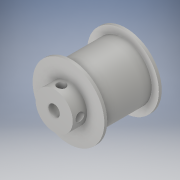
# Autodesk Inventor part: Timing Belt - 8mm Bore 5mm Pitch 14 Teeth 15mm Wide
Saved by Autodesk Inventor 2017 SP1 (Build 210196100, 196)
## iProperties
Created: 2017-10-06
Part Number: Timing Belt - 8mm Bore 5mm Pitch 14 Teeth 15mm Wide
Material: Aluminum 6061
Document SubType Name: Modeling
Designer: Zach
Density: 2.7 g/cm^3
Appearance: Aluminum - Flat
Author: Zach
Autodesk Inventor part; units mm, degrees
ref_plane "YZ Plane" through (0, 0, 0) normal (1, 0, 0) x (0, 1, 0)
ref_plane "XZ Plane" through (0, 0, 0) normal (0, 1, 0) x (-1, 0, 0)
ref_plane "XY Plane" through (0, 0, 0) normal (0, 0, 1) x (1, 0, 0)
sketch "Sketch1" plane through (0, 0, 0) normal (0, 0, 1) x (1, 0, 0)
  circle A0 centre (0, 0) radius 12.5
  circle A1 centre (0, 0) radius 2
  dimension "d0" = 25
  dimension "d1" = 4
  constraints: 2 centre point, 2 coincident
  measures "d0" diameter of A0
  measures "d1" diameter of A1
extrude "Extrusion1" add sketch "Sketch1" along normal blind 20
sketch "Sketch2" plane through (0, 0, 20) normal (0, 0, 1) x (1, 0, 0)
  circle A0 centre (0, 0) radius 2 projected
  circle A1 centre (0, 0) radius 6.5
  dimension "d4" = 13
  constraints: 1 centre point, 1 coincident
  measures "d4" diameter of A1
extrude "Extrusion2" add sketch "Sketch2" along normal blind 5
ref_plane "Work Plane1" through (0, 0, 10) normal (0, 0, -1) x (-1, 0, 0)
sketch "Sketch3" plane through (0, 0, 10) normal (0, 0, -1) x (-1, 0, 0)
  circle A0 centre (0, 0) radius 10
  circle A1 centre (0, 0) radius 12.5 projected
  dimension "d7" = 20
  constraints: 1 centre point, 1 coincident
  measures "d7" diameter of A0
extrude "Extrusion3" cut sketch "Sketch3" along normal mid plane 18
sketch "Sketch6" plane through (0, 0, 0) normal (0, 1, 0) x (-1, 0, 0)
  line L0 (6.5, 25) -> (-6.5, 25) projected
  line L1 (-6.5, 20) -> (6.5, 20) projected
  line L2 (-2, 25) -> (2, 25) projected
  line L3 (-2, 25) -> (2, 25) projected
  line L4 (2, 0) -> (-2, 0) projected
  circle A0 centre (0, 22.5) radius 1.5
  line L5 (6.5, 20) -> (6.5, 25) projected
  line L6 (-6.5, 20) -> (-6.5, 25) projected
  point P0 (0, 0)
  point P1 (0, 20)
  point P2 (6.5, 22.5)
  dimension "d36" = 3
  constraints: 2 midpoint, 1 centre point, 1 horizontal alignment, 1 vertical alignment
  measures "d36" diameter of A0
extrude "Extrusion4" cut sketch "Sketch6" along normal through all contours A0
sketch "Sketch7" plane through (0, 0, 0) normal (1, 0, 0) x (0, 1, 0)
  line L0 (-2, 25) -> (2, 25) projected
  line L1 (6.5, 20) -> (6.5, 25) projected
  circle A0 centre (0, 22.5) radius 1.5
  point P0 (0, 0)
  point P1 (0, 25)
  point P2 (6.5, 22.5)
  dimension "d39" = 3
  constraints: 2 midpoint, 1 centre point, 1 horizontal alignment, 1 vertical alignment
  measures "d39" diameter of A0
extrude "Extrusion5" cut sketch "Sketch7" along normal through all
body "Solid1"
